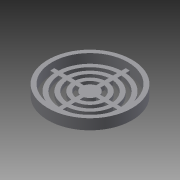
# Autodesk Inventor part: Lattice bottom
Saved by Autodesk Inventor 2013 (Build 170138000, 138)
## iProperties
Created: 2014-07-04
Part Number: Lattice bottom
Material: Genérico
Document SubType Name: Chapa
Designer: Administrador
Density: 1 g/cm^3
Sheet Metal Rule: Por defecto_mm
Author: Administrador
Autodesk Inventor part; units mm, degrees
ref_plane "YZ Plane" through (0, 0, 0) normal (1, 0, 0) x (0, 1, 0)
ref_plane "XZ Plane" through (0, 0, 0) normal (0, 1, 0) x (-1, 0, 0)
ref_plane "XY Plane" through (0, 0, 0) normal (0, 0, 1) x (1, 0, 0)
sketch "Boceto1" plane through (0, 0, 0) normal (0, 0, 1) x (1, 0, 0)
  circle A0 centre (0, 0) radius 20
  circle A1 centre (0, 0) radius 18
  dimension "d0" = 40
  dimension "d1" = 36
  constraints: 2 centre point
  measures "d0" diameter of A0
  measures "d1" diameter of A1
extrude "Extrusión1" add sketch "Boceto1" along normal blind 5
sketch "Boceto2" plane through (0, 0, 0) normal (0, 0, -1) x (-1, 0, 0)
  circle A0 centre (0, 0) radius 16
  circle A1 centre (0, 0) radius 14
  circle A2 centre (0, 0) radius 12
  circle A3 centre (0, 0) radius 10
  circle A4 centre (0, 0) radius 8
  circle A5 centre (0, 0) radius 6
  circle A6 centre (0, 0) radius 4
  dimension "d4" = 32
  dimension "d5" = 28
  dimension "d6" = 24
  dimension "d7" = 20
  dimension "d8" = 16
  dimension "d9" = 12
  dimension "d10" = 8
  constraints: 7 centre point
  measures "d4" diameter of A0
  measures "d5" diameter of A1
  measures "d6" diameter of A2
  measures "d7" diameter of A3
  measures "d8" diameter of A4
  measures "d9" diameter of A5
  measures "d10" diameter of A6
extrude "Extrusión2" add sketch "Boceto2" against normal blind 2
sketch "Boceto3" plane through (0, 0, 0) normal (0, 0, -1) x (-1, 0, 0)
  line L0 (-19.4045, 1) -> (19.4045, 1)
  line L1 (19.4045, 1) -> (19.4045, -1)
  line L2 (19.4045, -1) -> (-19.4045, -1)
  line L3 (-19.4045, -1) -> (-19.4045, 1)
  line L4 (-19.4045, 1) -> (19.4045, -1) construction
  line L5 (19.4045, 1) -> (-19.4045, -1) construction
  line L6 (-1, 19.4045) -> (1, 19.4045)
  line L7 (1, 19.4045) -> (1, -19.4045)
  line L8 (1, -19.4045) -> (-1, -19.4045)
  line L9 (-1, -19.4045) -> (-1, 19.4045)
  line L10 (-1, 19.4045) -> (1, -19.4045) construction
  line L11 (1, 19.4045) -> (-1, -19.4045) construction
  point P0 (0, 0)
  point P1 (0, 0)
  dimension "d13" = 2
  dimension "d14" = 2
  constraints: 24 end point, 4 midpoint, 4 parallel, 2 horizontal, 2 perpendicular
  measures "d13" distance of L0.end L1.end
  measures "d14" distance of L7.end L8.end
extrude "Extrusión3" add sketch "Boceto3" against normal blind 2
equation "\"Radio_pliegue\" = Grosor"
equation "\"Anchura_desahogo_plegado\" = Grosor"
equation "\"Profundidad_desahogo_plegado\" = 0.5 * Grosor"
equation "\"Tamaño_destalonado\" = 4 * Grosor"
equation "\"Remanente_mínimo\" = 2 * Grosor"
equation "\"Radiodetransición\" = Radio_pliegue"
equation "\"Tamaño_de_radio_de_Jacobi\" = Radio_pliegue"
equation "\"TamañoSeparación\" = Grosor"
equation "\"Grosor\" = 0.5"
